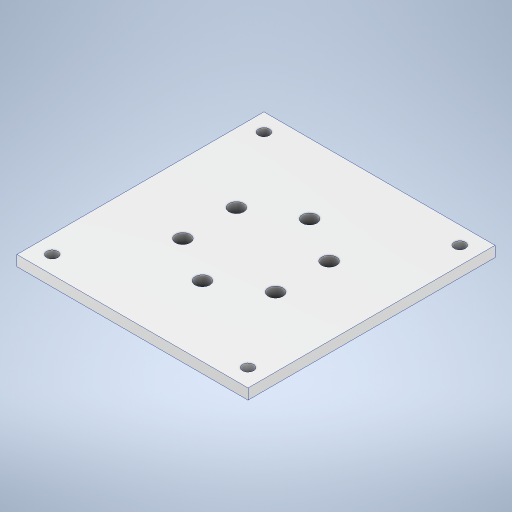
# Autodesk Inventor part: link2_plate4
Saved by Autodesk Inventor 2024 (Build 280153000, 153)
## iProperties
Created: 2024-12-13
Part Number: link2_plate4
Material: アルミニウム 6061
Document SubType Name: Modeling
Designer: hirek
Density: 2.7 g/cm^3
Appearance: アルミニウム - フラット
Author: hirek
Autodesk Inventor part; units mm, degrees
ref_plane "YZ Plane" through (0, 0, 0) normal (1, 0, 0) x (0, 1, 0)
ref_plane "XZ Plane" through (0, 0, 0) normal (0, 1, 0) x (-1, 0, 0)
ref_plane "XY Plane" through (0, 0, 0) normal (0, 0, 1) x (1, 0, 0)
sketch "スケッチ1" plane through (0, 0, 0) normal (0, 1, 0) x (-1, 0, 0)
  line L0 (0, 0) -> (65.5, 0)
  line L1 (65.5, 0) -> (65.5, -70)
  line L2 (65.5, -70) -> (0, -70)
  line L3 (0, -70) -> (0, 0)
  dimension "d0" = 65.5
  dimension "d1" = 70
  constraints: 8 end point, 2 parallel, 1 horizontal, 1 perpendicular
  measures "d0" distance of L1.end L2.end
  measures "d1" distance of L0.end L1.end
extrude "押し出し1" add sketch "スケッチ1" along normal blind 3
sketch "スケッチ2" plane through (0, 3, 0) normal (0, 1, 0) x (1, 0, 0)
  line L0 (-60.5, 5) -> (-5, 5)
  line L1 (-5, 5) -> (-5, 65)
  line L2 (-5, 65) -> (-60.5, 65)
  line L3 (-60.5, 65) -> (-60.5, 5)
  line L4 (-65.5, 0) -> (0, 0) projected
  line L5 (-65.5, 70) -> (-65.5, 0) projected
  dimension "d4" = 55.5
  dimension "d5" = 60
  dimension "d6" = 5
  dimension "d7" = 5
  constraints: 8 end point, 4 coincident, 2 parallel, 1 horizontal, 1 perpendicular
  measures "d4" distance of L2.end L1.end
  measures "d5" distance of L1.end L0.end
  measures "d6" distance between parallel lines of L0 L4
  measures "d7" distance between parallel lines of L5 L3
hole "穴1" at (-60.5, 3, -5) at (-5, 3, -5) at (-60.5, 3, -65) at (-5, 3, -65) direction (0, -1, 0) diameter 3.2 end through all
sketch "スケッチ3" plane through (0, 3, 0) normal (0, 1, 0) x (1, 0, 0)
  line L0 (-65.5, 0) -> (0, 0) projected
  line L1 (-32.75, 0) -> (-32.75, 70)
  line L2 (0, 70) -> (-65.5, 70) projected
  circle A0 centre (-32.75, 35) radius 15.18
  line L3 (0, 70) -> (-65.5, 70) projected
  line L4 (-65.5, 70) -> (-65.5, 0) projected
  point P0 (-32.75, 50.18)
  point P1 (-45.8963, 42.59)
  point P2 (-45.8963, 27.41)
  point P3 (-32.75, 19.82)
  point P4 (-19.6037, 27.41)
  point P5 (-19.6037, 42.59)
  dimension "d15" = 30.36
  dimension "d18" = 360
  dimension "d27" = 32.75
  constraints: 2 end point, 1 midpoint, 1 perpendicular, 1 point on line, 1 vertical alignment, 9 other
  measures "d27" distance between parallel lines of L1 L4
hole "穴2" at (-32.75, 3, -50.18) at (-45.8963, 3, -42.59) at (-45.8963, 3, -27.41) at (-32.75, 3, -19.82) at (-19.6037, 3, -27.41) at (-19.6037, 3, -42.59) direction (0, -1, 0) diameter 4.2 end through all
